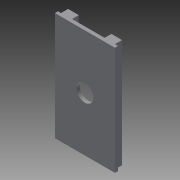
# Autodesk Inventor part: adapter-slot
Saved by Autodesk Inventor 2015 (Build 190159000, 159)
## iProperties
Created: 2014-07-18
Part Number: adapter-slot
Material: Generic
Document SubType Name: Modeling
Designer: pc
Density: 1 g/cm^3
Appearance: Default
Author: pc
Autodesk Inventor part; units mm, degrees
ref_plane "YZ Plane" through (0, 0, 0) normal (1, 0, 0) x (0, 1, 0)
ref_plane "XZ Plane" through (0, 0, 0) normal (0, 1, 0) x (-1, 0, 0)
ref_plane "XY Plane" through (0, 0, 0) normal (0, 0, 1) x (1, 0, 0)
sketch "Sketch1" plane through (0, 0, 0) normal (0, 1, 0) x (-1, 0, 0)
  line L0 (7.95, 15.98) -> (-7.95, 15.98)
  line L1 (-7.95, 15.98) -> (-7.95, -15.98)
  line L2 (-7.95, -15.98) -> (7.95, -15.98)
  line L3 (7.95, -15.98) -> (7.95, 15.98)
  line L4 (7.95, 15.98) -> (-7.95, -15.98) construction
  line L5 (-7.95, 15.98) -> (7.95, -15.98) construction
  point P0 (0, 0)
  dimension "d0" = 31.96
  dimension "d1" = 15.9
  constraints: 12 end point, 2 midpoint, 2 parallel, 1 horizontal, 1 perpendicular
  measures "d0" distance of L0.end L1.end
  measures "d1" distance of L0.start L0.end
extrude "adapter-arm" add sketch "Sketch1" along normal blind 3
sketch "fanslot" plane through (0, 3, 0) normal (0, 1, 0) x (1, 0, 0)
  line L0 (-4.8, -15.98) -> (4.8, -15.98)
  line L1 (4.8, -15.98) -> (5.5, 15.98)
  line L2 (5.5, 15.98) -> (-5.5, 15.98)
  line L3 (-5.5, 15.98) -> (-4.8, -15.98)
  line L4 (0, 16.157) -> (0, -15.9695) construction
  line L5 (-7.95, -15.98) -> (7.95, -15.98) construction
  line L6 (7.95, 15.98) -> (-7.95, 15.98) construction
  point P0 (0, 0)
  point P1 (0, -15.98)
  point P2 (0, 15.98)
  point P3 (-5.98, -15.98)
  point P4 (5.98, -15.98)
  point P5 (5.98, 15.98)
  point P6 (-5.98, 15.98)
  dimension "d21" = 11
  dimension "d22" = 9.6
  constraints: 10 end point, 3 point on line, 2 collinear, 2 midpoint, 1 horizontal, 1 parallel, 1 vertical
  measures "d21" distance of L1.end L2.end
  measures "d22" distance of L0.start L0.end
extrude "Extrusion3" cut sketch "fanslot" against normal blind 2
sketch "Sketch5" plane through (0, 0, 0) normal (0, -1, 0) x (1, 0, 0)
  circle A0 centre (0, 0) radius 2.5
  dimension "d25" = 5
  constraints: 1 centre point, 1 coincident
  measures "d25" diameter of A0
extrude "Extrusion4" cut sketch "Sketch5" against normal up to next
sketch "Sketch6" plane through (-7.95, 0, 15.98) normal (0, 0, 1) x (1, 0, 0)
  line L0 (0, 0) -> (-0.9, 0)
  line L1 (-0.9, 0) -> (-0.9, 0.9)
  line L2 (-0.9, 0.9) -> (0, 0.9)
  line L3 (0, 0.9) -> (0, 0)
  line L4 (15.9, 0) -> (16.8, 0)
  line L5 (16.8, 0) -> (16.8, 0.9)
  line L6 (16.8, 0.9) -> (15.9, 0.9)
  line L7 (15.9, 0.9) -> (15.9, 0)
  point P0 (7.95, 0)
  dimension "d28" = 0.9
  dimension "d29" = 0.9
  dimension "d30" = 0.9
  dimension "d31" = 0.9
  constraints: 16 end point, 4 parallel, 2 horizontal, 2 perpendicular
  measures "d28" distance of L1.end L2.end
  measures "d29" distance of L0.end L1.end
  measures "d30" distance of L6.end L5.end
  measures "d31" distance of L5.end L4.end
extrude "Extrusion5" add sketch "Sketch6" against normal up to surface (31.96 mm away)
equation "\"d2\" = armthick"
equation "\"d21\" = fanhb"
equation "\"d22\" = fanhs"
equation "\"d23\" = armslotd"
equation "\"printer3dtolerance\" = 0.12"
equation "\"wallw\" = 42"
equation "\"wallh\" = 44"
equation "\"cornerrad\" = 2"
equation "\"baseextra\" = 2"
equation "\"wall1_thick\" = 8"
equation "\"wall2_thick\" = 6.4"
equation "\"wall3_thick\" = 4"
equation "\"wall1slot\" = 8.12"
equation "\"wall2slot\" = 6.52"
equation "\"wall3slot\" = 4.12"
equation "\"gap2\" = 28"
equation "\"baseh\" = 79.12"
equation "\"basew\" = 44"
equation "\"base_thick\" = 6"
equation "\"base_slots_depth\" = 4"
equation "\"servobigcircledia\" = 11.62"
equation "\"servosmallcircledia\" = 5.92"
equation "\"servo9gw\" = 22.8"
equation "\"servomounth\" = 4"
equation "\"servomountsquare\" = 4"
equation "\"servopolygonr\" = 6.12"
equation "\"servopolygonl\" = 5.92"
equation "\"distancefrombottom\" = 34"
equation "\"distancefromleft\" = 22"
equation "\"wall3slotd\" = 2"
equation "\"wall3slotw\" = 36"
equation "\"adapterh\" = 16"
equation "\"adapterw\" = 32"
equation "\"armw\" = 34"
equation "\"armslotd\" = 2"
equation "\"armthick\" = 3"
equation "\"fanhb\" = 11"
equation "\"fanhs\" = 9.6"
equation "\"adapterwallthick\" = 6"
equation "\"adapterwallslotd\" = 2"
equation "\"hornscrewheadd\" = 3"
equation "\"hornscrewholed\" = 2"
equation "\"hornthick\" = 1.5"
equation "\"armhornthick\" = 3"
body "Solid1"
